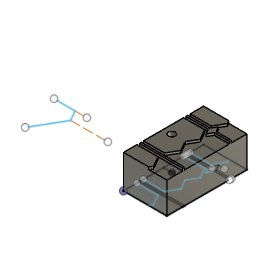
Biegelehre_LED v4 (Autodesk Fusion 360 design; units mm, degrees)
Autodesk Fusion 360 part; units mm, degrees
sketch "Skizze1" plane through (0, 0, 0) normal (0, 0, 1) x (1, 0, 0)
  line L0 (0, 0) -> (26, 0)
  line L1 (26, 0) -> (26, 48)
  line L2 (26, 48) -> (0, 48)
  line L3 (0, 48) -> (0, 0)
  line L4 (-68.6314, 26.9805) -> (-56.0314, 26.9805)
  line L5 (-56.0314, 26.9805) -> (-52.4314, 20.7451)
  line L6 (-56.0314, 26.9805) -> (-48.9309, 26.9805) construction
  line L7 (-52.4314, 20.7451) -> (-62.4314, 3.4246)
  line L8 (-52.4314, 20.7451) -> (-30.1306, 20.7451) construction
  line L9 (0, 10.58) -> (26, 10.58)
  line L10 (26, 10.58) -> (26, 9.42)
  line L11 (26, 9.42) -> (0, 9.42)
  line L12 (0, 9.42) -> (0, 10.58)
  line L13 (0, 8.04) -> (12.6, 8.04)
  line L14 (12.6, 8.04) -> (16.2, 1.8046)
  line L15 (16.2, 1.8046) -> (15.1581, 0)
  line L16 (0, 11.96) -> (12.6, 11.96)
  line L17 (12.6, 11.96) -> (16.2, 18.1954)
  line L18 (16.2, 18.1954) -> (12.8487, 24)
  line L19 (0, 36.04) -> (12.6, 36.04)
  line L20 (12.6, 36.04) -> (16.2, 29.8046)
  line L21 (16.2, 29.8046) -> (12.8487, 24)
  line L22 (16.2, 46.1954) -> (15.1581, 48)
  line L23 (12.6, 39.96) -> (16.2, 46.1954)
  line L24 (0, 39.96) -> (12.6, 39.96)
  line L25 (13.4, 38.58) -> (15.2, 41.6977)
  line L26 (13.4, 38.58) -> (14.4685, 38.58) construction
  line L27 (15.2, 41.6977) -> (17, 38.58)
  line L28 (15.2, 41.6977) -> (18.8, 41.6977) construction
  line L29 (13.4, 37.42) -> (15.2, 34.3023)
  line L30 (15.2, 34.3023) -> (17, 37.42)
  line L31 (26, 37.42) -> (17, 37.42)
  line L32 (13.4, 37.42) -> (0, 37.42)
  line L33 (0, 38.58) -> (13.4, 38.58)
  line L34 (17, 38.58) -> (26, 38.58)
  line L35 (0, 24) -> (5, 24)
  circle A0 centre (5, 24) radius 1.25
  dimension "d1" = 26
  dimension "d2" = 48
  dimension "d3" = 12.6
  dimension "d4" = 7.2
  dimension "d5" = 60
  dimension "d6" = 120
  dimension "d7" = 20
  dimension "d8" = 1.16
  dimension "d13" = 12.6
  dimension "d14" = 7.2
  dimension "d16" = 12.6
  dimension "d17" = 7.2
  dimension "d19" = 1.16
  dimension "d20" = 13.4
  dimension "d21" = 3.6
  dimension "d22" = 60
  dimension "d23" = 60
  dimension "d24" = 3.6
  dimension "d26" = 28
  dimension "d28" = 9.42
  dimension "d33" = 5
  dimension "d34" = 24
  dimension "d35" = 2.5
  constraint horizontal L0
  constraint vertical L1
  constraint horizontal L2
  constraint vertical L3
  constraint coincident L0.start L3.end
  constraint horizontal L4
  constraint horizontal L6
  constraint horizontal L8
  constraint horizontal L9
  constraint vertical L10
  constraint horizontal L11
  constraint vertical L12
  constraint coincident L1 L10.end
  constraint coincident L3 L9.start
  constraint horizontal L13
  constraint horizontal L19
  constraint horizontal L33
  constraint horizontal L31
  constraint coincident L0 L15.end
  constraint coincident L2 L22.end
  constraint horizontal L26
  constraint horizontal L28
  constraint collinear L31 L32
  constraint collinear L33 L34
  constraint coincident L3 L35.start
  constraint perpendicular L3 L35
  constraint coincident L35.end A0.centre
  measures "d1" distance of L0.start L0.end
  measures "d2" distance of L0.start L2.end
  measures "d3" distance of L4.start L4.end
  measures "d4" distance of L4.end L5.end
  measures "d5" angle of L5 L6
  measures "d6" angle of L7 L8
  measures "d7" distance of L5.end L7.end
  measures "d8" distance of L9 L11
  measures "d13" distance of L13.start L13.end
  measures "d14" distance of L14.end L13.end
  measures "d16" distance of L19.start L19.end
  measures "d17" distance of L20.end L19.end
  measures "d19" distance of L31 L33
  measures "d20" distance of L3 L25.start
  measures "d21" distance of L25.start L25.end
  measures "d22" angle of L25 L26
  measures "d23" angle of L27 L28
  measures "d24" distance of L25.end L27.end
  measures "d26" distance of L9 L33
  measures "d28" distance of L0 L11
  measures "d33" distance of L35.start L35.end
  measures "d34" distance of L0 L35
  measures "d35" diameter of A0
extrude "Extrusion3" add sketch "Skizze1" along normal blind 20 contours L0 L3 L13 L14 L15 | L1 L3 L9 L10 L11 L12 | L3 L16 L17 L18 L19 L20 L21 | L1 L3 L25 L27 L29 L30 L31 L32 L33 L34 | L2 L3 L22 L23 L24 makes body 1 at (0, 28.0133, 6.6667) makes body 2 at (8.9333, 37.42, 6.6667) makes body 3 at (8.6667, 10.58, 6.6667) makes body 4 at (10.1054, 48, 6.6667) makes body 5 at (5.0527, 0, 6.6667)
extrude "Extrusion4" add sketch "Skizze1" along normal blind 18.6 contours L0 L1 L3 L11 L13 L14 L15 | L1 L3 L9 L16 L17 L18 L19 L20 L21 L29 L30 L31 L32 | L1 L2 L3 L22 L23 L24 L25 L27 L33 L34 bodies 1 2 3 4 5
chamfer "Fase1" distance 0.8 distance2 2 1 edges at (3.8346, 24.452, 20) measured on face at (5.9594, 32.4329, 20) on bodies 1
chamfer "Fase2" distance 2 distance2 0.8 1 edges at (3.8346, 24.452, 0) measured on face at (6.2438, 24.1245, 6) on bodies 1
